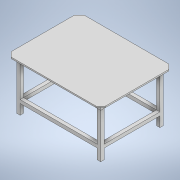
# Autodesk Inventor part: Mesa_Centrado
Saved by Autodesk Inventor 2021 (Build 250183000, 183)
## iProperties
Created: 2021-06-07
Part Number: Mesa_Centrado
Material: Genérico
Document SubType Name: Modeling
Designer: Mecatronica
Density: 1 g/cm^3
Appearance: Valor por defecto
Author: Mecatronica
Autodesk Inventor part; units mm, degrees
ref_plane "YZ Plane" through (0, 0, 0) normal (1, 0, 0) x (0, 1, 0)
ref_plane "XZ Plane" through (0, 0, 0) normal (0, 1, 0) x (-1, 0, 0)
sketch "Boceto1" plane through (0, 0, 0) normal (0, 1, 0) x (-1, 0, 0)
  line L0 (692.5, 535) -> (-692.5, 535)
  line L1 (-692.5, 535) -> (-692.5, -535)
  line L2 (-692.5, -535) -> (692.5, -535)
  line L3 (692.5, -535) -> (692.5, 535)
  line L4 (622.5, 535) -> (692.5, 465)
  line L5 (692.5, 0) -> (-692.5, 0)
  line L6 (0, 535) -> (0, -535)
  line L7 (622.5, -535) -> (692.5, -465)
  line L8 (-622.5, 535) -> (-692.5, 465)
  line L9 (-622.5, -535) -> (-692.5, -465)
  point P0 (0, 0)
  point P1 (-622.5, 535)
  point P2 (-692.5, 465)
  point P3 (-692.5, -465)
  point P4 (-622.5, -535)
  point P5 (622.5, -535)
  point P6 (692.5, -465)
  dimension "d0" = 1070
  dimension "d1" = 1385
  dimension "d2" = 692.5
  dimension "d3" = 535
  dimension "d4" = 70
  dimension "d5" = 70
  constraints: 20 end point, 6 symmetric about line, 4 midpoint, 2 parallel, 2 point on line, 1 horizontal, 1 perpendicular
  measures "d0" distance of L2.end L0.start
  measures "d1" distance of L0.start L0.end
  measures "d2" distance from line of point (0, 0) L3
  measures "d3" distance from line of point (0, 0) L2
  measures "d4" distance of L4.end L0.start
  measures "d5" distance of L4.start L0.start
extrude "Extrusión1" add sketch "Boceto1" along normal blind 20 contours L4 L3 L5 L6 L0 | L6 L5 L1 L8 L0 | L3 L7 L2 L6 L5 | L6 L2 L9 L1 L5
sketch "Boceto2" plane through (0, 0, 0) normal (0, -1, 0) x (1, 0, 0)
  line L0 (-642.5, 485) -> (642.5, 485)
  line L1 (642.5, 485) -> (642.5, -485)
  line L2 (642.5, -485) -> (-642.5, -485)
  line L3 (-642.5, -485) -> (-642.5, 485)
  line L4 (-622.5, 535) -> (622.5, 535) projected
  line L5 (-692.5, -465) -> (-692.5, 465) projected
  line L6 (622.5, -535) -> (-622.5, -535) projected
  line L7 (692.5, 465) -> (692.5, -465) projected
  line L8 (-617.5, 460) -> (617.5, 460)
  line L9 (617.5, 460) -> (617.5, -460)
  line L10 (617.5, -460) -> (-617.5, -460)
  line L11 (-617.5, -460) -> (-617.5, 460)
  point P0 (0, 0)
  dimension "d8" = 50
  dimension "d9" = 50
  dimension "d10" = 50
  dimension "d11" = 50
  dimension "d12" = 25
  dimension "d13" = 25
  dimension "d14" = 25
  dimension "d15" = 25
  constraints: 16 end point, 4 parallel, 2 horizontal, 2 perpendicular
  measures "d8" distance between parallel lines of L4 L0
  measures "d9" distance between parallel lines of L3 L5
  measures "d10" distance between parallel lines of L6 L2
  measures "d11" distance between parallel lines of L7 L1
  measures "d12" distance between parallel lines of L0 L8
  measures "d13" distance between parallel lines of L3 L11
  measures "d14" distance between parallel lines of L2 L10
  measures "d15" distance between parallel lines of L1 L9
extrude "Extrusión2" add sketch "Boceto2" along normal blind 50
sketch "Boceto3" plane through (0, 0, 0) normal (0, -1, 0) x (1, 0, 0)
  line L0 (-617.5, 460) -> (617.5, 460) projected
  line L1 (-617.5, 460) -> (-567.5, 460)
  line L2 (-567.5, 460) -> (-567.5, 410)
  line L3 (-567.5, 410) -> (-617.5, 410)
  line L4 (-617.5, 410) -> (-617.5, 460)
  line L5 (0, 460) -> (0, -460)
  line L6 (617.5, -460) -> (-617.5, -460) projected
  line L7 (-617.5, 460) -> (-617.5, -460) projected
  line L8 (-617.5, 0) -> (472.5, 0)
  line L9 (617.5, 460) -> (567.5, 460)
  line L10 (567.5, 460) -> (567.5, 410)
  line L11 (567.5, 410) -> (617.5, 410)
  line L12 (617.5, 410) -> (617.5, 460)
  line L13 (-617.5, -460) -> (-567.5, -460)
  line L14 (-567.5, -460) -> (-567.5, -410)
  line L15 (-567.5, -410) -> (-617.5, -410)
  line L16 (-617.5, -410) -> (-617.5, -460)
  line L17 (617.5, -460) -> (567.5, -460)
  line L18 (567.5, -460) -> (567.5, -410)
  line L19 (567.5, -410) -> (617.5, -410)
  line L20 (617.5, -410) -> (617.5, -460)
  point P0 (0, 0)
  point P1 (567.5, 460)
  point P2 (567.5, -460)
  point P3 (-617.5, -410)
  point P4 (-567.5, -460)
  dimension "d18" = 50
  dimension "d19" = 50
  constraints: 36 end point, 9 symmetric about line, 3 midpoint, 2 horizontal, 2 parallel, 1 perpendicular
  measures "d18" distance of L1.end L2.end
  measures "d19" distance of L2.end L3.end
extrude "Extrusión3" add sketch "Boceto3" along normal blind 730 contours L0 L12 L11 L10 | L18 L19 L20 L6 | L0 L2 L3 L4 | L15 L14 L6 L7
sketch "Boceto4" plane through (-617.5, -50, 460) normal (0, 0, 1) x (1, 0, 0)
  line L0 (0, 0) -> (0, -680) projected
  line L1 (0, -530) -> (50, -530)
  line L2 (50, 0) -> (50, -680) projected
  line L3 (50, -680) -> (0, -680) projected
  point P0 (617.5, 50)
  dimension "d23" = 150
  constraints: 2 end point, 2 point on line, 1 horizontal
  measures "d23" distance between parallel lines of L1 L3
sketch "Boceto5" plane through (567.5, 0, -410) normal (0, 0, 1) x (1, 0, 0)
  line L0 (0, -50) -> (0, -730) projected
  line L1 (0, -580) -> (50, -580)
  line L2 (50, -50) -> (50, -730) projected
  line L3 (50, -730) -> (0, -730) projected
  point P0 (-567.5, 0)
  dimension "d24" = 150
  constraints: 2 end point, 2 point on line, 1 horizontal
  measures "d24" distance between parallel lines of L1 L3
ref_plane "Plano de trabajo2" through (-617.5, -580, 460) normal (0, 1, 0) x (1, 0, 0)
sketch "Boceto6" plane through (-617.5, -580, 460) normal (0, 1, 0) x (1, 0, 0)
  line L0 (0, 0) -> (50, 0) projected
  line L1 (1235, 50) -> (1185, 50) projected
  line L2 (50, 0) -> (1185, 0)
  line L3 (1185, 0) -> (1185, 50)
  line L4 (1185, 50) -> (50, 50)
  line L5 (50, 50) -> (50, 0)
  line L6 (1185, 50) -> (1185, 0) projected
  line L7 (1235, 50) -> (1235, 870) projected
  line L8 (1185, 50) -> (1235, 50)
  line L9 (1235, 50) -> (1235, 870)
  line L10 (1235, 870) -> (1185, 870)
  line L11 (1185, 870) -> (1185, 50)
  line L12 (1185, 920) -> (1185, 870) projected
  line L13 (50, 870) -> (50, 920) projected
  line L14 (1185, 870) -> (50, 870)
  line L15 (50, 870) -> (50, 920)
  line L16 (50, 920) -> (1185, 920)
  line L17 (1185, 920) -> (1185, 870)
  line L18 (0, 870) -> (0, 50) projected
  line L19 (50, 870) -> (0, 870)
  line L20 (0, 870) -> (0, 50)
  line L21 (0, 50) -> (50, 50)
  line L22 (50, 50) -> (50, 870)
  point P0 (617.5, 460)
  point P1 (50, 50)
  point P2 (50, 50)
  point P3 (50, 870)
  point P4 (50, 870)
  point P5 (0, 870)
  constraints: 32 end point, 8 parallel, 4 horizontal, 4 perpendicular
extrude "Extrusión4" add sketch "Boceto6" along normal blind 50 contours L1 L11 L10 L7 | L3 L2 L5 L4 | L21 L18 L19 L22 | L14 L13 L16 L12
equation "\"d2\" = 0.5 * d1"
equation "\"d3\" = 0.5 * d0"
equation "\"d9\" = d8"
equation "\"d10\" = d8"
equation "\"d11\" = d9"
equation "\"d13\" = d12"
equation "\"d14\" = d12"
equation "\"d15\" = d12"
equation "\"d18\" = d19"
